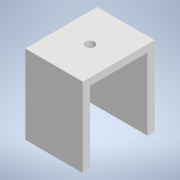
# Autodesk Inventor part: brazo
Saved by Autodesk Inventor 2020.3 (Build 243373000, 373)
## iProperties
Created: 2021-01-29
Part Number: brazo
Material: Generic
Document SubType Name: Modeling
Designer: Yu Jinyu
Density: 1 g/cm^3
Appearance: Default
Author: Yu Jinyu
Autodesk Inventor part; units mm, degrees
ref_plane "YZ Plane" through (0, 0, 0) normal (1, 0, 0) x (0, 1, 0)
ref_plane "XZ Plane" through (0, 0, 0) normal (0, 1, 0) x (-1, 0, 0)
ref_plane "XY Plane" through (0, 0, 0) normal (0, 0, 1) x (1, 0, 0)
sketch "Sketch1" plane through (0, 0, 0) normal (0, 0, 1) x (1, 0, 0)
  line L0 (-10, -25) -> (10, -25)
  line L1 (10, -25) -> (10, 25)
  line L2 (10, 25) -> (-10, 25)
  line L3 (-10, 25) -> (-10, -25)
  line L4 (-10, -25) -> (10, 25) construction
  line L5 (10, -25) -> (-10, 25) construction
  point P0 (0, 0)
  dimension "d0" = 20
  dimension "d1" = 50
  constraints: 12 end point, 2 midpoint, 2 parallel, 1 horizontal, 1 perpendicular
  measures "d0" distance of L2.end L1.end
  measures "d1" distance of L1.end L0.end
ref_plane "Work Plane1" through (-10, 25, 0) normal (0, 1, 0) x (1, 0, 0)
sketch "Sketch2" plane through (-10, 25, 0) normal (0, 1, 0) x (1, 0, 0)
  line L0 (20, 0) -> (0, 0) projected
  line L1 (0, 0) -> (20, 0)
  line L2 (20, 0) -> (20, -40)
  line L3 (20, -40) -> (0, -40)
  line L4 (0, -40) -> (0, 0)
  point P0 (10, 0)
  dimension "d4" = 40
  constraints: 8 end point, 2 parallel, 1 horizontal, 1 perpendicular
  measures "d4" distance of L1.end L2.end
extrude "Extrusion2" add sketch "Sketch2" along normal blind 5
sketch "Sketch3" plane through (-10, 25, 40) normal (0, 0, 1) x (1, 0, 0)
  line L0 (20, -50) -> (20, 0) projected
  line L1 (20, 0) -> (0, 0) projected
  line L2 (0, 0) -> (0, -50) projected
  line L3 (0, -50) -> (20, -50) projected
  line L4 (0, 0) -> (20, 0) projected
  line L5 (20, 0) -> (20, 5) projected
  line L6 (0, 5) -> (20, 5) projected
  line L7 (0, 0) -> (0, 5) projected
  point P0 (10, -25)
extrude "Extrusion3" add sketch "Sketch3" along normal blind 5
extrude "Extrusion4" add sketch "Sketch1" against normal blind 5
sketch "Sketch4" plane through (10, 30, 0) normal (0, 0, -1) x (-1, 0, 0)
  line L0 (0, -5) -> (20, -5) projected
  line L1 (20, -5) -> (20, 0) projected
  line L2 (0, 0) -> (20, 0) projected
  line L3 (0, -5) -> (0, 0) projected
  point P0 (10, -30)
extrude "Extrusion5" add sketch "Sketch4" along normal blind 5
sketch "Sketch5" plane through (-10, 30, 0) normal (0, 1, 0) x (1, 0, 0)
  circle A0 centre (10, -20) radius 2.6
  point P0 (10, 0)
  dimension "d13" = 5.2
  constraints: 1 centre point
  measures "d13" diameter of A0
extrude "Extrusion6" cut sketch "Sketch5" against normal blind 10
sketch "Sketch6" plane through (-10, 30, 0) normal (0, 1, 0) x (1, 0, 0)
  line L0 (20, 0) -> (20, 5) projected
  line L1 (20, 5) -> (30, 5)
  line L2 (30, 5) -> (30, -45)
  line L3 (30, -45) -> (20, -45)
  line L4 (20, -45) -> (20, 5)
  line L5 (20, 5) -> (0, 5) projected
  line L6 (0, 5) -> (-10, 5)
  line L7 (-10, 5) -> (-10, -45)
  line L8 (-10, -45) -> (0, -45)
  line L9 (0, -45) -> (0, 5)
  point P0 (10, 0)
  dimension "d16" = 10
  dimension "d17" = 50
  dimension "d18" = 10
  constraints: 16 end point, 4 parallel, 2 horizontal, 2 perpendicular, 1 point on line
  measures "d16" distance of L2.end L3.end
  measures "d17" distance of L1.end L2.end
  measures "d18" distance of L8.end L7.end
extrude "Extrusion7" add sketch "Sketch6" against normal blind 5
sketch "Sketch7" plane through (-10, 25, 0) normal (0, -1, 0) x (1, 0, 0)
  line L0 (20, -5) -> (30, -5) projected
  line L1 (30, -5) -> (20, -5)
  line L2 (20, -5) -> (20, 0)
  line L3 (20, 0) -> (30, 0)
  line L4 (30, 0) -> (30, -5)
  line L5 (30, -5) -> (-10, -5) projected
  line L6 (0, 0) -> (0, -5) projected
  line L7 (-10, -5) -> (0, -5)
  line L8 (0, -5) -> (0, 0)
  line L9 (0, 0) -> (-10, 0)
  line L10 (-10, 0) -> (-10, -5)
  line L11 (-10, 45) -> (30, 45) projected
  line L12 (30, -5) -> (30, 45) projected
  line L13 (20, 45) -> (30, 45)
  line L14 (30, 45) -> (30, 40)
  line L15 (30, 40) -> (20, 40)
  line L16 (20, 40) -> (20, 45)
  line L17 (-10, 45) -> (0, 45)
  line L18 (0, 45) -> (0, 40)
  line L19 (0, 40) -> (-10, 40)
  line L20 (-10, 40) -> (-10, 45)
  point P0 (10, 0)
  dimension "d21" = 5
  constraints: 32 end point, 8 parallel, 4 horizontal, 4 perpendicular, 3 point on line
  measures "d21" distance of L13.end L14.end
extrude "Extrusion8" add sketch "Sketch7" along normal blind 50
body "Solid1"
